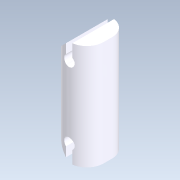
# Autodesk Inventor part: ring_f1
Saved by Autodesk Inventor 2020.2 (Build 242310000, 310)
## iProperties
Created: 2020-05-30
Part Number: ring_f1
Material: Generic
Document SubType Name: Modeling
Designer: Bardo91
Density: 1 g/cm^3
Appearance: Default
Author: Bardo91
Autodesk Inventor part; units mm, degrees
ref_plane "YZ Plane" through (0, 0, 0) normal (1, 0, 0) x (0, 1, 0)
ref_plane "XZ Plane" through (0, 0, 0) normal (0, 1, 0) x (-1, 0, 0)
ref_plane "XY Plane" through (0, 0, 0) normal (0, 0, 1) x (1, 0, 0)
sketch "Sketch1" plane through (0, 0, 0) normal (0, 0, 1) x (1, 0, 0)
  line L0 (0, 0) -> (2.5, 0)
  line L1 (2.5, 0) -> (2.5, 50)
  line L2 (2.5, 50) -> (-2.5, 50)
  line L3 (-2.5, 50) -> (-2.5, 0)
  circle A0 centre (0, 0) radius 8.5
  line L4 (0, 50) -> (8.5, 50) construction
  circle A1 centre (0, 50) radius 8.5
  line L5 (-8.5, 0) -> (-8.5, 50)
  line L6 (8.5, 50) -> (8.5, 0)
  line L7 (0, 50) -> (8.5, 50)
  line L8 (0, 50) -> (-8.5, 41.5)
  line L9 (0, 50) -> (12.0208, 50) construction
  line L10 (0, 0) -> (8.5, 0)
  line L11 (0, 0) -> (-8.5, 8.5)
  line L12 (0, 0) -> (12.0208, 0) construction
  dimension "d9" = 17
  dimension "d1" = 2.5
  dimension "d2" = 50
  dimension "d3" = 5
  dimension "d5" = 17
  dimension "d10" = 2.5
  dimension "d11" = 0
  dimension "d12" = 135
  dimension "d13" = 135
  constraints: 26 end point, 4 horizontal, 3 coincident, 3 perpendicular, 3 point on line, 2 equal length, 2 point on circle, 2 tangent, 2 vertical, 1 centre point, 1 collinear, 1 horizontal alignment, 2 other
  measures "d1" distance of L0.start L0.end
  measures "d2" distance of L0.end L1.end
  measures "d3" distance of L1.end L2.end
  measures "d5" diameter of A0
  measures "d10" distance from line of L3 L4.start
  measures "d11" distance from line of L2 L4.start
  measures "d12" angle of L8 L9
  measures "d13" angle of L12 L11
extrude "Extrusion1" add sketch "Sketch1" along normal blind 20 contours L11 L3 A0 L1 L0 | L1 A0 L10 | L11 A0 L3 | A0 L3 A1 L1 | L1 A1 L6 A0 | A0 L11 L5 L8 A1 L3 | A1 L3 L8 L2 L1 | L1 L7 A1 | A1 L8 L3
sketch "Sketch2" plane through (0, 0, 0) normal (0, 0, -1) x (-1, 0, 0)
  line L0 (0, 0) -> (-8.5, 0) projected
  line L1 (0, 0) -> (0, 8)
  circle A0 centre (0, 8) radius 2.5
  line L2 (8.5, 8.5) -> (0, 0) projected
  line L3 (0, 0) -> (-1.5, 0)
  line L4 (-1.5, 0) -> (-1.5, 8)
  line L5 (-1.5, 8) -> (1.5, 8)
  line L6 (1.5, 8) -> (1.5, 0)
  line L7 (1.5, 0) -> (0, 0)
  line L8 (0, 50) -> (8.5, 41.5) projected
  line L9 (0, 50) -> (0, 42)
  line L10 (0, 42) -> (-1.5, 42)
  line L11 (-1.5, 42) -> (-1.5, 50)
  line L12 (-8.5, 50) -> (0, 50) projected
  line L13 (0, 42) -> (1.5, 42)
  line L14 (1.5, 42) -> (1.5, 50)
  line L15 (1.5, 50) -> (0, 50)
  circle A1 centre (0, 42) radius 2.5
  point P0 (1.5, 45)
  point P1 (-1.5, 44)
  point P2 (1.5, 44)
  point P3 (-1.5, 6)
  point P4 (1.5, 6)
  dimension "d16" = 8
  dimension "d17" = 5
  dimension "d18" = 1.5
  dimension "d19" = 3
  dimension "d20" = 8
  dimension "d21" = 1.5
  dimension "d22" = 1.5
  dimension "d23" = 5
  constraints: 24 end point, 7 point on line, 4 perpendicular, 2 centre point, 2 coincident, 2 vertical, 1 collinear
  measures "d16" distance of L0.start L1.end
  measures "d17" diameter of A0
  measures "d18" distance of L0.start L3.end
  measures "d19" distance of L4.end L5.end
  measures "d20" distance of L8.start L9.end
  measures "d21" distance of L9.end L10.end
  measures "d22" distance of L9.end L13.end
  measures "d23" diameter of A1
extrude "Extrusion2" cut sketch "Sketch2" against normal through all
fillet "Fillet1" radius 8 4 edges at (8.5, 25, 0) (8.5, 25, 20) (-8.5, 25, 0) (-8.5, 25, 20)
sketch "Sketch4" plane through (1.5, 0, 0.0627) normal (0, -1, 0) x (1, 0, 0)
  line L0 (-10, 7.9373) -> (-10, 11.9373) projected
  line L1 (-10, 9.9373) -> (-8, 9.9373)
  circle A0 centre (-8, 9.9373) radius 1
  point P0 (-1.5, -0.0627)
  dimension "d31" = 2
  dimension "d32" = 2
  constraints: 2 end point, 1 centre point, 1 coincident, 1 horizontal, 1 midpoint
  measures "d31" distance of L1.start L1.end
  measures "d32" diameter of A0
extrude "Extrusion4" cut sketch "Sketch4" against normal through all
body "Solid1"
